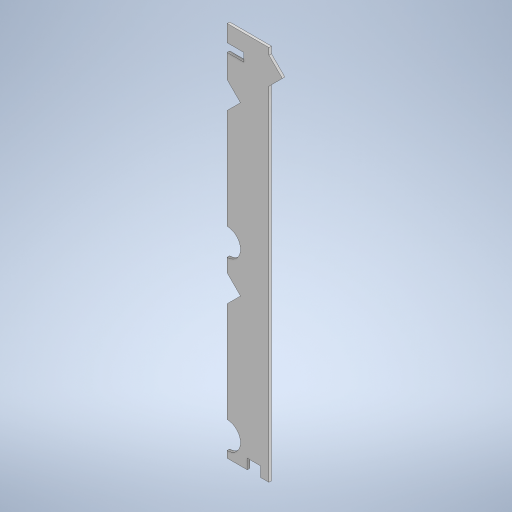
# Autodesk Inventor part: MS_FI_v3
Saved by Autodesk Inventor 2024 (Build 280153000, 153)
## iProperties
Created: 2023-03-29
Part Number: MS_FI_v3
Material: Generic
Document SubType Name: Modeling
Designer: LKLM8608
Density: 1 g/cm^3
Appearance: Default
Author: LKLM8608
Autodesk Inventor part; units mm, degrees
ref_plane "YZ Plane" through (0, 0, 0) normal (1, 0, 0) x (0, 1, 0)
ref_plane "XZ Plane" through (0, 0, 0) normal (0, 1, 0) x (-1, 0, 0)
ref_plane "XY Plane" through (0, 0, 0) normal (0, 0, 1) x (1, 0, 0)
sketch "Sketch1" plane through (0, 0, 0) normal (0, 0, 1) x (1, 0, 0)
  circle A0 centre (0, 213.2) radius 8 construction
  line L0 (0, 221.2) -> (8, 213.2)
  line L1 (0, 205.2) -> (8, 213.2)
  line L2 (0, 0) -> (0, 205.2)
  line L3 (0, 225.2) -> (-25, 225.2)
  line L4 (-25, 0) -> (-13, 0)
  line L5 (-13, 0) -> (-13, 6)
  line L6 (-13, 6) -> (-5, 6)
  line L7 (-5, 6) -> (-5, 0)
  line L8 (-25, 0) -> (-13, 0)
  line L9 (-5, 0) -> (0, 0)
  line L10 (-25, 196.1) -> (-17, 188.1)
  line L11 (-17, 188.1) -> (-25, 180.1)
  arc A1 (-25, 104.1) -> (-25, 120.1) centre (-25, 112.1) ccw
  line L12 (-25, 180.1) -> (-25, 120.1)
  circle A2 centre (-25, 188.1) radius 8 construction
  line L13 (0, 221.2) -> (0, 225.2)
  line L14 (-25, 215.2) -> (-15, 215.2)
  line L15 (-15, 215.2) -> (-15, 210.2)
  line L16 (-15, 210.2) -> (-25, 210.2)
  line L17 (-25, 225.2) -> (-25, 215.2)
  line L18 (-25, 210.2) -> (-25, 196.1)
  arc A3 (-25, 4) -> (-25, 20) centre (-25, 12) ccw
  line L19 (-25, 4) -> (-25, 0)
  line L20 (-25, 96) -> (-17, 88)
  line L21 (-17, 88) -> (-25, 80)
  circle A4 centre (-25, 88) radius 8 construction
  line L22 (-25, 104.1) -> (-25, 96)
  line L23 (-25, 80) -> (-25, 20)
  dimension "d5" = 16
  dimension "d168" = 25
  dimension "d177" = 12
  dimension "d178" = 6
  dimension "d179" = 8
  dimension "d189" = 76
  dimension "d193" = 4
  dimension "d194" = 10
  dimension "d195" = 5
  dimension "d196" = 225.2
  dimension "d197" = 10
  dimension "d198" = 37.1
  dimension "d199" = 76
  dimension "d200" = 24.1
  dimension "d201" = 5
  constraints: 48 end point, 30 perpendicular, 11 point on circle, 7 vertical alignment, 6 collinear, 5 centre point, 4 equal radius, 2 horizontal, 2 horizontal alignment, 1 coincident, 1 vertical
  measures "d5" diameter of A0
  measures "d168" distance of L4.start L2.start
  measures "d177" distance of L4.start L4.end
  measures "d178" distance of L4.end L5.end
  measures "d179" distance of L5.end L6.end
  measures "d189" distance of A1.centre A2.centre
  measures "d193" distance of L3.start L0.start
  measures "d194" distance of L14.start L14.end
  measures "d195" distance of L14.end L15.end
  measures "d196" distance between parallel lines of L9 L3
  measures "d197" distance between parallel lines of L3 L14
  measures "d198" distance from line of L3 A2.centre
  measures "d199" distance of A3.centre A4.centre
  measures "d200" distance of A4.centre A1.centre
  measures "d201" distance between parallel lines of L2 L7
extrude "Extrusion10" add sketch "Sketch1" along normal blind 1.5
body "Solid2"
